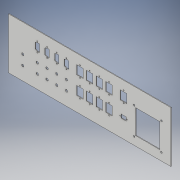
# Autodesk Inventor part: PDU_chassis
Saved by Autodesk Inventor 2017 (Build 210142000, 142)
## iProperties
Created: 2017-02-13
Part Number: PDU_chassis
Material: Generic
Document SubType Name: Modeling
Designer: Zara
Density: 1 g/cm^3
Appearance: Default
Author: Zara
Autodesk Inventor part; units mm, degrees
ref_plane "YZ Plane" through (0, 0, 0) normal (1, 0, 0) x (0, 1, 0)
ref_plane "XZ Plane" through (0, 0, 0) normal (0, 1, 0) x (-1, 0, 0)
ref_plane "XY Plane" through (0, 0, 0) normal (0, 0, 1) x (1, 0, 0)
sketch "Sketch1" plane through (0, 0, 0) normal (0, 0, 1) x (1, 0, 0)
  line L0 (-212.471, -66.7512) -> (212.471, -66.7512)
  line L1 (212.471, -66.7512) -> (212.471, 66.7512)
  line L2 (212.471, 66.7512) -> (-212.471, 66.7512)
  line L3 (-212.471, 66.7512) -> (-212.471, -66.7512)
  line L4 (-212.471, -66.7512) -> (212.471, 66.7512) construction
  line L5 (212.471, -66.7512) -> (-212.471, 66.7512) construction
  point P0 (0, 0)
  dimension "d0" = 424.942
  dimension "d1" = 133.5024
  constraints: 12 end point, 2 midpoint, 2 parallel, 1 horizontal, 1 perpendicular
  measures "d0" distance of L1.end L2.end
  measures "d1" distance of L0.end L1.end
extrude "pdu" add sketch "Sketch1" along normal blind 1.651
sketch "dsub9 sketch" plane through (0, 0, 1.651) normal (0, 0, 1) x (1, 0, 0)
  line L0 (-137.033, 41.9354) -> (-137.033, 16.9418) construction
  line L1 (-127.711, 29.4386) -> (-146.355, 29.4386) construction
  circle A0 centre (-137.033, 16.9418) radius 1.1303
  circle A1 centre (-137.033, 41.9354) radius 1.1303
  line L2 (-131.191, 37.8733) -> (-131.191, 21.0039)
  line L3 (-142.875, 36.1061) -> (-142.875, 22.7711)
  arc A2 (-133.7847, 18.9524) -> (-131.191, 21.0039) centre (-133.2992, 21.0039) ccw
  arc A3 (-142.875, 22.7711) -> (-141.2523, 20.7196) centre (-140.7668, 22.7711) ccw
  arc A4 (-141.1558, 38.1781) -> (-142.875, 36.1061) centre (-140.7668, 36.1061) ccw
  arc A5 (-131.191, 37.1546) -> (-133.6574, 39.5859) centre (-133.2684, 37.5139) ccw
  line L4 (-133.6574, 39.5859) -> (-141.1558, 38.1781)
  line L5 (-133.7847, 18.9524) -> (-141.2523, 20.7196)
  line L6 (209.423, 58.4962) -> (-209.423, 58.4962) construction
  line L7 (-209.423, 58.4962) -> (-209.423, -58.4962) construction
  line L8 (-209.423, -58.4962) -> (209.423, -58.4962) construction
  line L9 (209.423, -58.4962) -> (209.423, 58.4962) construction
  line L10 (212.471, 66.7512) -> (-212.471, 66.7512) construction
  line L11 (-212.471, -66.7512) -> (212.471, -66.7512) construction
  line L12 (-212.471, 66.7512) -> (-212.471, -66.7512) construction
  line L13 (212.471, -66.7512) -> (212.471, 66.7512) construction
  line L14 (-133.2992, 18.8957) -> (-149.9459, 18.8957) construction
  line L15 (-108.2574, 39.5859) -> (-115.7558, 38.1781)
  arc A6 (-105.791, 37.1546) -> (-108.2574, 39.5859) centre (-107.8684, 37.5139) ccw
  line L16 (-102.311, 29.4386) -> (-120.955, 29.4386) construction
  line L17 (-108.3847, 18.9524) -> (-115.8523, 20.7196)
  line L18 (-105.791, 37.8733) -> (-105.791, 21.0039)
  line L19 (-107.8992, 18.8957) -> (-124.5459, 18.8957) construction
  circle A7 centre (-111.633, 16.9418) radius 1.1303
  arc A8 (-108.3847, 18.9524) -> (-105.791, 21.0039) centre (-107.8992, 21.0039) ccw
  line L20 (-117.475, 36.1061) -> (-117.475, 22.7711)
  arc A9 (-117.475, 22.7711) -> (-115.8523, 20.7196) centre (-115.3668, 22.7711) ccw
  line L21 (-111.633, 41.9354) -> (-111.633, 16.9418) construction
  circle A10 centre (-111.633, 41.9354) radius 1.1303
  arc A11 (-115.7558, 38.1781) -> (-117.475, 36.1061) centre (-115.3668, 36.1061) ccw
  line L22 (-82.8574, 39.5859) -> (-90.3558, 38.1781)
  arc A12 (-80.391, 37.1546) -> (-82.8574, 39.5859) centre (-82.4684, 37.5139) ccw
  line L23 (-76.911, 29.4386) -> (-95.555, 29.4386) construction
  line L24 (-82.9847, 18.9524) -> (-90.4523, 20.7196)
  line L25 (-80.391, 37.8733) -> (-80.391, 21.0039)
  line L26 (-82.4992, 18.8957) -> (-99.1459, 18.8957) construction
  circle A13 centre (-86.233, 16.9418) radius 1.1303
  arc A14 (-82.9847, 18.9524) -> (-80.391, 21.0039) centre (-82.4992, 21.0039) ccw
  line L27 (-92.075, 36.1061) -> (-92.075, 22.7711)
  arc A15 (-92.075, 22.7711) -> (-90.4523, 20.7196) centre (-89.9668, 22.7711) ccw
  line L28 (-86.233, 41.9354) -> (-86.233, 16.9418) construction
  circle A16 centre (-86.233, 41.9354) radius 1.1303
  arc A17 (-90.3558, 38.1781) -> (-92.075, 36.1061) centre (-89.9668, 36.1061) ccw
  line L29 (-57.4574, 39.5859) -> (-64.9558, 38.1781)
  arc A18 (-54.991, 37.1546) -> (-57.4574, 39.5859) centre (-57.0684, 37.5139) ccw
  line L30 (-51.511, 29.4386) -> (-70.155, 29.4386) construction
  line L31 (-57.5847, 18.9524) -> (-65.0523, 20.7196)
  line L32 (-54.991, 37.8733) -> (-54.991, 21.0039)
  line L33 (-57.0992, 18.8957) -> (-73.7459, 18.8957) construction
  circle A19 centre (-60.833, 16.9418) radius 1.1303
  arc A20 (-57.5847, 18.9524) -> (-54.991, 21.0039) centre (-57.0992, 21.0039) ccw
  line L34 (-66.675, 36.1061) -> (-66.675, 22.7711)
  arc A21 (-66.675, 22.7711) -> (-65.0523, 20.7196) centre (-64.5668, 22.7711) ccw
  line L35 (-60.833, 41.9354) -> (-60.833, 16.9418) construction
  circle A22 centre (-60.833, 41.9354) radius 1.1303
  arc A23 (-64.9558, 38.1781) -> (-66.675, 36.1061) centre (-64.5668, 36.1061) ccw
  point P0 (0, 0)
  point P1 (-137.033, 29.4386)
  point P2 (-131.191, 29.4386)
  point P3 (-142.875, 29.4386)
  point P4 (-105.791, 29.4386)
  point P5 (-111.633, 29.4386)
  point P6 (-117.475, 29.4386)
  point P7 (-80.391, 29.4386)
  point P8 (-86.233, 29.4386)
  point P9 (-92.075, 29.4386)
  point P10 (-54.991, 29.4386)
  point P11 (-60.833, 29.4386)
  point P12 (-66.675, 29.4386)
  dimension "d24" = 38.1
  dimension "d205" = 25.4
  dimension "d208" = 25.4
  dimension "d4" = 2.2606
  dimension "d5" = 2.2606
  dimension "d6" = 24.9936
  dimension "d7" = 4.2164
  dimension "d8" = 4.2164
  dimension "d9" = 4.2164
  dimension "d10" = 4.2164
  dimension "d11" = 13.335
  dimension "d12" = 16.51
  dimension "d13" = 8.255
  dimension "d14" = 8.255
  dimension "d15" = 3.048
  dimension "d16" = 3.048
  dimension "d17" = 75.438
  dimension "d18" = 5.842
  dimension "d19" = 11.684
  dimension "d21" = 7.4985
  dimension "d165" = 37.3126
  dimension "d175" = 25.4
  constraints: 64 end point, 40 point on circle, 24 centre point, 12 point on line, 8 coincident, 8 tangent, 5 horizontal, 4 midpoint, 3 vertical, 2 parallel, 1 collinear, 1 perpendicular, 110 other
  measures "d4" diameter of A1
  measures "d5" diameter of A0
  measures "d6" distance of L0.start L0.end
  measures "d7" diameter of A2
  measures "d8" diameter of A3
  measures "d9" diameter of A5
  measures "d10" diameter of A4
  measures "d11" distance of A3.centre A4.centre
  measures "d12" distance of A2.centre A5.centre
  measures "d13" distance between parallel lines of L10 L6
  measures "d14" distance between parallel lines of L11 L8
  measures "d15" distance between parallel lines of L12 L7
  measures "d16" distance between parallel lines of L13 L9
  measures "d17" distance from line of L12 A0.centre
  measures "d18" distance from line of L2 A0.centre
  measures "d19" distance between parallel lines of L3 L2
  measures "d21" horizontal distance of A4.centre A5.centre
  measures "d165" distance between parallel lines of L10 L1
  measures "d175" distance of A4.centre A11.centre
sketch "CAT7 sketch" plane through (0, 0, 1.651) normal (0, 0, 1) x (1, 0, 0)
  line L0 (-34.124, 40.8686) -> (-16.979, 40.8686)
  line L1 (-16.979, 40.8686) -> (-16.979, 18.0086)
  line L2 (-16.979, 18.0086) -> (-34.124, 18.0086)
  line L3 (-34.124, 18.0086) -> (-34.124, 40.8686)
  line L4 (-43.4069, 29.4386) -> (12.6608, 29.4386) construction
  circle A0 centre (-25.5515, 43.942) radius 1.1303
  circle A1 centre (-25.5515, 14.9352) radius 1.1303
  line L5 (-25.5515, 43.942) -> (-25.5515, 14.9352) construction
  line L6 (-212.471, -66.7512) -> (212.471, -66.7512) construction
  line L7 (-212.471, 66.7512) -> (-212.471, -66.7512) construction
  line L8 (-34.124, -6.1722) -> (-16.979, -6.1722)
  line L9 (-16.979, -6.1722) -> (-16.979, -29.0322)
  line L10 (-16.979, -29.0322) -> (-34.124, -29.0322)
  line L11 (-34.124, -29.0322) -> (-34.124, -6.1722)
  circle A2 centre (-25.5515, -3.1073) radius 1.1303
  circle A3 centre (-25.5515, -32.1141) radius 1.1303
  line L12 (-25.5515, -3.1073) -> (-25.5515, -32.1141) construction
  circle A4 centre (-0.1515, 14.9352) radius 1.1303
  line L13 (8.421, 18.0086) -> (-8.724, 18.0086)
  line L14 (-18.0069, 29.4386) -> (38.0608, 29.4386) construction
  line L15 (8.421, 40.8686) -> (8.421, 18.0086)
  line L16 (-8.724, 40.8686) -> (8.421, 40.8686)
  line L17 (-8.724, 18.0086) -> (-8.724, 40.8686)
  line L18 (-0.1515, 43.942) -> (-0.1515, 14.9352) construction
  circle A5 centre (-0.1515, 43.942) radius 1.1303
  circle A6 centre (-0.1515, -3.1073) radius 1.1303
  line L19 (-8.724, -6.1722) -> (8.421, -6.1722)
  line L20 (8.421, -6.1722) -> (8.421, -29.0322)
  line L21 (8.421, -29.0322) -> (-8.724, -29.0322)
  line L22 (-8.724, -29.0322) -> (-8.724, -6.1722)
  line L23 (-0.1515, -3.1073) -> (-0.1515, -32.1141) construction
  circle A7 centre (-0.1515, -32.1141) radius 1.1303
  circle A8 centre (25.2485, 14.9352) radius 1.1303
  line L24 (33.821, 18.0086) -> (16.676, 18.0086)
  line L25 (7.3931, 29.4386) -> (63.4608, 29.4386) construction
  line L26 (33.821, 40.8686) -> (33.821, 18.0086)
  line L27 (16.676, 40.8686) -> (33.821, 40.8686)
  line L28 (16.676, 18.0086) -> (16.676, 40.8686)
  line L29 (25.2485, 43.942) -> (25.2485, 14.9352) construction
  circle A9 centre (25.2485, 43.942) radius 1.1303
  circle A10 centre (25.2485, -3.1073) radius 1.1303
  line L30 (16.676, -6.1722) -> (33.821, -6.1722)
  line L31 (33.821, -6.1722) -> (33.821, -29.0322)
  line L32 (33.821, -29.0322) -> (16.676, -29.0322)
  line L33 (16.676, -29.0322) -> (16.676, -6.1722)
  line L34 (25.2485, -3.1073) -> (25.2485, -32.1141) construction
  circle A11 centre (25.2485, -32.1141) radius 1.1303
  circle A12 centre (50.6485, 14.9352) radius 1.1303
  line L35 (59.221, 18.0086) -> (42.076, 18.0086)
  line L36 (32.7931, 29.4386) -> (88.8608, 29.4386) construction
  line L37 (59.221, 40.8686) -> (59.221, 18.0086)
  line L38 (42.076, 40.8686) -> (59.221, 40.8686)
  line L39 (42.076, 18.0086) -> (42.076, 40.8686)
  line L40 (50.6485, 43.942) -> (50.6485, 14.9352) construction
  circle A13 centre (50.6485, 43.942) radius 1.1303
  circle A14 centre (50.6485, -3.1073) radius 1.1303
  line L41 (42.076, -6.1722) -> (59.221, -6.1722)
  line L42 (59.221, -6.1722) -> (59.221, -29.0322)
  line L43 (59.221, -29.0322) -> (42.076, -29.0322)
  line L44 (42.076, -29.0322) -> (42.076, -6.1722)
  line L45 (50.6485, -3.1073) -> (50.6485, -32.1141) construction
  circle A15 centre (50.6485, -32.1141) radius 1.1303
  line L46 (32.9446, 29.4386) -> (89.0123, 29.4386) construction
  line L47 (80.176, 40.8686) -> (97.321, 40.8686)
  line L48 (97.321, 40.8686) -> (97.321, 18.0086)
  line L49 (97.321, 18.0086) -> (80.176, 18.0086)
  line L50 (80.176, 18.0086) -> (80.176, 40.8686)
  circle A16 centre (88.7485, 43.942) radius 1.1303
  circle A17 centre (88.7485, 14.9352) radius 1.1303
  line L51 (88.7485, 43.942) -> (88.7485, 14.9352) construction
  line L52 (212.471, 66.7512) -> (-212.471, 66.7512) projected
  line L53 (40.3437, -17.6022) -> (62.8778, -17.6022) construction
  point P0 (0, 0)
  point P1 (-34.124, 29.4386)
  point P2 (-25.5515, 40.8686)
  point P3 (-25.5515, 29.4386)
  point P4 (-25.5515, -6.1807)
  point P5 (-34.124, -17.6107)
  point P6 (-43.4069, -17.6107)
  point P7 (-25.5515, -17.6107)
  point P8 (25.4, 0)
  point P9 (-8.724, 29.4386)
  point P10 (-0.1515, 29.4386)
  point P11 (-0.1515, 40.8686)
  point P12 (-0.1515, -6.1807)
  point P13 (-18.0069, -17.6107)
  point P14 (-0.1515, -17.6107)
  point P15 (-8.724, -17.6107)
  point P16 (50.8, 0)
  point P17 (16.676, 29.4386)
  point P18 (25.2485, 29.4386)
  point P19 (25.2485, 40.8686)
  point P20 (25.2485, -6.1807)
  point P21 (7.3931, -17.6107)
  point P22 (25.2485, -17.6107)
  point P23 (16.676, -17.6107)
  point P24 (76.2, 0)
  point P25 (42.076, 29.4386)
  point P26 (50.6485, 29.4386)
  point P27 (50.6485, 40.8686)
  point P28 (50.6485, -6.1807)
  point P29 (32.7931, -17.6107)
  point P30 (50.6485, -17.6107)
  point P31 (42.076, -17.6107)
  point P32 (80.176, 29.4386)
  point P33 (88.7485, 40.8686)
  point P34 (88.7485, 29.4386)
  point P35 (98.2853, 29.4386)
  dimension "d47" = 22.86
  dimension "d48" = 17.145
  dimension "d49" = 2.2606
  dimension "d50" = 2.2606
  dimension "d51" = 29.0068
  dimension "d52" = 81.6864
  dimension "d53" = 186.9195
  dimension "d56" = 47.0408
  dimension "d132" = 25.4
  dimension "d146" = 22.86
  dimension "d147" = 17.145
  dimension "d148" = 2.2606
  dimension "d149" = 2.2606
  dimension "d150" = 29.0068
  dimension "d151" = 38.1
  dimension "d152" = 25.8826
  constraints: 94 end point, 18 centre point, 17 point on line, 8 horizontal, 6 midpoint, 4 parallel, 3 vertical, 2 perpendicular, 1 collinear, 119 other
  measures "d47" distance of L0.end L1.end
  measures "d48" distance of L1.end L2.end
  measures "d49" diameter of A0
  measures "d50" diameter of A1
  measures "d51" distance of L5.end L5.start
  measures "d52" distance from line of L6 L5.end
  measures "d53" distance from line of L7 L5.end
  measures "d56" distance of L0.start L11.end
  measures "d132" distance of point (0, 0) point (25.4, 0)
  measures "d146" distance of L47.end L49.start
  measures "d147" distance of L49.start L50.start
  measures "d148" diameter of A16
  measures "d149" diameter of A17
  measures "d150" distance of L51.end L51.start
  measures "d151" distance from line of L40 point (88.748, 29.439)
  measures "d152" distance between parallel lines of L52 L47
sketch "Sketch5" plane through (0, 0, 1.651) normal (0, 0, 1) x (1, 0, 0)
  line L0 (110.109, -53.1622) -> (193.929, -53.1622) construction
  line L1 (193.929, -53.1622) -> (193.929, 30.6578) construction
  line L2 (193.929, 30.6578) -> (110.109, 30.6578) construction
  line L3 (110.109, 30.6578) -> (110.109, -53.1622) construction
  line L4 (110.109, -53.1622) -> (193.929, 30.6578) construction
  line L5 (193.929, -53.1622) -> (110.109, 30.6578) construction
  line L6 (-212.471, 66.7512) -> (-212.471, -66.7512) projected
  line L7 (-212.471, -66.7512) -> (212.471, -66.7512) projected
  line L8 (120.269, -43.0022) -> (183.769, -43.0022)
  line L9 (183.769, -43.0022) -> (183.769, 20.4978)
  line L10 (183.769, 20.4978) -> (120.269, 20.4978)
  line L11 (120.269, 20.4978) -> (120.269, -43.0022)
  line L12 (120.269, -43.0022) -> (183.769, 20.4978) construction
  line L13 (183.769, -43.0022) -> (120.269, 20.4978) construction
  line L14 (116.332, -46.9392) -> (187.706, -46.9392) construction
  line L15 (187.706, -46.9392) -> (187.706, 24.4348) construction
  line L16 (187.706, 24.4348) -> (116.332, 24.4348) construction
  line L17 (116.332, 24.4348) -> (116.332, -46.9392) construction
  line L18 (116.332, -46.9392) -> (187.706, 24.4348) construction
  line L19 (187.706, -46.9392) -> (116.332, 24.4348) construction
  circle A0 centre (116.332, 24.4348) radius 2.2479
  circle A1 centre (187.706, 24.4348) radius 2.2479
  circle A2 centre (187.706, -46.9392) radius 2.2479
  circle A3 centre (116.332, -46.9392) radius 2.2479
  line L20 (120.269, -43.0022) -> (183.769, -43.0022)
  line L21 (183.769, -43.0022) -> (183.769, 20.4978)
  line L22 (183.769, 20.4978) -> (120.269, 20.4978)
  line L23 (120.269, 20.4978) -> (120.269, -43.0022)
  line L24 (120.269, -43.0022) -> (183.769, 20.4978) construction
  line L25 (183.769, -43.0022) -> (120.269, 20.4978) construction
  point P0 (0, 0)
  point P1 (152.019, -11.2522)
  point P2 (152.019, -11.2522)
  dimension "d63" = 83.82
  dimension "d64" = 83.82
  dimension "d65" = 322.58
  dimension "d66" = 13.589
  dimension "d67" = 63.5
  dimension "d68" = 63.5
  dimension "d69" = 71.374
  dimension "d70" = 4.4958
  dimension "d71" = 4.4958
  dimension "d72" = 4.4958
  dimension "d73" = 4.4958
  constraints: 48 end point, 10 midpoint, 8 parallel, 4 centre point, 4 horizontal, 4 perpendicular, 3 coincident, 1 point on line
  measures "d63" distance of L1.end L2.end
  measures "d64" distance of L2.end L0.start
  measures "d65" distance between parallel lines of L6 L3
  measures "d66" distance between parallel lines of L0 L7
  measures "d67" distance of L8.end L9.end
  measures "d68" distance of L8.start L8.end
  measures "d69" distance of L14.start L14.end
  measures "d70" diameter of A1
  measures "d71" diameter of A0
  measures "d72" diameter of A2
  measures "d73" diameter of A3
hole "airflow holes" at (187.706, 24.4348, 1.651) at (116.332, 24.4348, 1.651) at (116.332, -46.9392, 1.651) at (187.706, -46.9392, 1.651) direction (0, 0, -1) diameter 4.4958 end through all clearance for "Flat Head Machine Screw (82)" size "#8" standard "Ansi Unified Screw Threads"
sketch "Sketch7" plane through (0, 0, 1.651) normal (0, 0, 1) x (1, 0, 0)
  line L0 (110.109, -53.1622) -> (193.929, -53.1622) construction
  line L1 (193.929, -53.1622) -> (193.929, 30.6578) construction
  line L2 (193.929, 30.6578) -> (110.109, 30.6578) construction
  line L3 (110.109, 30.6578) -> (110.109, -53.1622) construction
  line L4 (110.109, -53.1622) -> (193.929, 30.6578) construction
  line L5 (193.929, -53.1622) -> (110.109, 30.6578) construction
  line L6 (-212.471, 66.7512) -> (-212.471, -66.7512)
  line L7 (-212.471, -66.7512) -> (212.471, -66.7512)
  line L8 (120.269, -43.0022) -> (183.769, -43.0022)
  line L9 (183.769, -43.0022) -> (183.769, 20.4978)
  line L10 (183.769, 20.4978) -> (120.269, 20.4978)
  line L11 (120.269, 20.4978) -> (120.269, -43.0022)
  line L12 (120.269, -43.0022) -> (183.769, 20.4978) construction
  line L13 (183.769, -43.0022) -> (120.269, 20.4978) construction
  line L14 (116.332, -46.9392) -> (187.706, -46.9392) construction
  line L15 (187.706, -46.9392) -> (187.706, 24.4348) construction
  line L16 (187.706, 24.4348) -> (116.332, 24.4348) construction
  line L17 (116.332, 24.4348) -> (116.332, -46.9392) construction
  line L18 (116.332, -46.9392) -> (187.706, 24.4348) construction
  line L19 (187.706, -46.9392) -> (116.332, 24.4348) construction
  circle A0 centre (116.332, 24.4348) radius 2.2479
  circle A1 centre (187.706, 24.4348) radius 2.2479
  circle A2 centre (187.706, -46.9392) radius 2.2479
  circle A3 centre (116.332, -46.9392) radius 2.2479
  line L20 (120.269, -43.0022) -> (183.769, -43.0022)
  line L21 (183.769, -43.0022) -> (183.769, 20.4978)
  line L22 (183.769, 20.4978) -> (120.269, 20.4978)
  line L23 (120.269, 20.4978) -> (120.269, -43.0022)
  line L24 (120.269, -43.0022) -> (183.769, 20.4978) construction
  line L25 (183.769, -43.0022) -> (120.269, 20.4978) construction
  point P0 (0, 0)
  point P1 (0, 0)
  point P2 (152.019, -11.2522)
  point P3 (152.019, -11.2522)
  dimension "d83" = 83.82
  dimension "d84" = 83.82
  dimension "d85" = 322.58
  dimension "d86" = 13.589
  dimension "d87" = 63.5
  dimension "d88" = 63.5
  dimension "d89" = 71.374
  dimension "d90" = 4.4958
  dimension "d91" = 4.4958
  dimension "d92" = 4.4958
  dimension "d93" = 4.4958
  constraints: 52 end point, 10 midpoint, 8 parallel, 4 centre point, 4 horizontal, 4 perpendicular, 3 coincident, 1 point on line
  measures "d83" distance of L1.end L2.end
  measures "d84" distance of L2.end L0.start
  measures "d85" distance between parallel lines of L6 L3
  measures "d86" distance between parallel lines of L0 L7
  measures "d87" distance of L8.end L9.end
  measures "d88" distance of L8.start L8.end
  measures "d89" distance of L14.start L14.end
  measures "d90" diameter of A1
  measures "d91" diameter of A0
  measures "d92" diameter of A2
  measures "d93" diameter of A3
extrude "airflow cutout" cut sketch "Sketch7" against normal through all contours L11 L10 L9 L8
hole "CAT7 holes" at (-25.5515, 43.942, 1.651) at (-25.5515, 14.9352, 1.651) at (-25.5515, -3.1073, 1.651) at (-25.5515, -32.1141, 1.651) at (-0.1515, 43.942, 1.651) at (-0.1515, 14.9352, 1.651) at (25.2485, 43.942, 1.651) at (25.2485, 14.9352, 1.651) at (50.6485, 43.942, 1.651) at (50.6485, 14.9352, 1.651) at (-0.1515, -3.1073, 1.651) at (-0.1515, -32.1141, 1.651) at (25.2485, -32.1141, 1.651) at (25.2485, -3.1073, 1.651) at (50.6485, -3.1073, 1.651) at (50.6485, -32.1141, 1.651) at (88.7485, 43.942, 1.651) at (88.7485, 14.9352, 1.651) direction (0, 0, -1) diameter 2.9464 end through all
extrude "CAT7 cutout" cut sketch "CAT7 sketch" against normal through all contours L0 L1 L2 L3 | L8 L9 L10 L11 | L13 L17 L16 L15 | L19 L20 L21 L22 | L24 L28 L27 L26 | L30 L31 L32 L33 | L35 L39 L38 L37 | L41 L42 L43 L44 | L47 L48 L49 L50
sketch "sma" plane through (0, 0, 1.651) normal (0, 0, 1) x (1, 0, 0)
  line L0 (-175.126, 2.9121) -> (-175.126, -16.382) construction
  line L1 (-183.1756, -6.2272) -> (-164.6712, -6.2272) construction
  arc A0 (-177.92, -7.7352) -> (-177.92, -4.7191) centre (-175.126, -6.2272) ccw
  line L2 (-177.92, -4.7191) -> (-177.92, -7.7352)
  line L3 (-137.033, 41.9354) -> (-137.033, 16.9418) construction
  line L4 (-137.026, 2.9121) -> (-137.026, -16.382) construction
  arc A1 (-139.82, -7.7352) -> (-139.82, -4.7191) centre (-137.026, -6.2272) ccw
  line L5 (-139.82, -4.7191) -> (-139.82, -7.7352)
  line L6 (-145.0756, -6.2272) -> (-126.5712, -6.2272) construction
  line L7 (-175.126, -22.4879) -> (-175.126, -41.782) construction
  arc A2 (-177.92, -33.1352) -> (-177.92, -30.1191) centre (-175.126, -31.6272) ccw
  line L8 (-177.92, -30.1191) -> (-177.92, -33.1352)
  line L9 (-183.1756, -31.6272) -> (-164.6712, -31.6272) construction
  line L10 (-137.026, -22.4879) -> (-137.026, -41.782) construction
  arc A3 (-139.82, -33.1352) -> (-139.82, -30.1191) centre (-137.026, -31.6272) ccw
  line L11 (-139.82, -30.1191) -> (-139.82, -33.1352)
  line L12 (-145.0756, -31.6272) -> (-126.5712, -31.6272) construction
  line L13 (-111.626, -22.4879) -> (-111.626, -41.782) construction
  line L14 (-114.42, -30.1191) -> (-114.42, -33.1352)
  arc A4 (-114.42, -33.1352) -> (-114.42, -30.1191) centre (-111.626, -31.6272) ccw
  line L15 (-114.42, -4.7191) -> (-114.42, -7.7352)
  line L16 (-119.6756, -31.6272) -> (-101.1712, -31.6272) construction
  arc A5 (-114.42, -7.7352) -> (-114.42, -4.7191) centre (-111.626, -6.2272) ccw
  line L17 (-119.6756, -6.2272) -> (-101.1712, -6.2272) construction
  line L18 (-86.226, -22.4879) -> (-86.226, -41.782) construction
  line L19 (-89.02, -30.1191) -> (-89.02, -33.1352)
  arc A6 (-89.02, -33.1352) -> (-89.02, -30.1191) centre (-86.226, -31.6272) ccw
  line L20 (-89.02, -4.7191) -> (-89.02, -7.7352)
  line L21 (-94.2756, -31.6272) -> (-75.7712, -31.6272) construction
  arc A7 (-89.02, -7.7352) -> (-89.02, -4.7191) centre (-86.226, -6.2272) ccw
  line L22 (-94.2756, -6.2272) -> (-75.7712, -6.2272) construction
  line L23 (-60.826, -22.4879) -> (-60.826, -41.782) construction
  line L24 (-63.62, -30.1191) -> (-63.62, -33.1352)
  arc A8 (-63.62, -33.1352) -> (-63.62, -30.1191) centre (-60.826, -31.6272) ccw
  line L25 (-63.62, -4.7191) -> (-63.62, -7.7352)
  line L26 (-68.8756, -31.6272) -> (-50.3712, -31.6272) construction
  arc A9 (-63.62, -7.7352) -> (-63.62, -4.7191) centre (-60.826, -6.2272) ccw
  line L27 (-68.8756, -6.2272) -> (-50.3712, -6.2272) construction
  point P0 (0, 0)
  point P1 (-171.951, -6.2272)
  point P2 (-133.851, -6.2272)
  point P3 (-171.951, -31.6272)
  point P4 (-133.851, -31.6272)
  point P5 (-108.451, -31.6272)
  point P6 (-111.626, -16.382)
  point P7 (-108.451, -6.2272)
  point P8 (-83.051, -31.6272)
  point P9 (-86.226, -16.382)
  point P10 (-83.051, -6.2272)
  point P11 (-57.651, -31.6272)
  point P12 (-60.826, -16.382)
  point P13 (-57.651, -6.2272)
  dimension "d208" = 25.4
  dimension "d123" = 6.35
  dimension "d124" = 5.969
  dimension "d191" = 38.1
  dimension "d198" = 25.4
  dimension "d205" = 25.4
  constraints: 54 end point, 30 point on circle, 27 point on line, 10 centre point, 3 collinear, 3 horizontal, 3 vertical, 99 other
  measures "d123" diameter of A0
  measures "d124" distance from line of point (-171.951, -6.227) L2
  measures "d191" distance of L0.start L4.start
  measures "d198" distance of L0.start L7.start
  measures "d205" distance of L12.start L16.start
extrude "sma cutouts" cut sketch "sma" against normal through all
sketch "sc/sc" plane through (0, 0, 1.651) normal (0, 0, 1) x (1, 0, 0)
  line L0 (82.0175, -12.9032) -> (95.4795, -12.9032)
  line L1 (95.4795, -12.9032) -> (95.4795, -22.3012)
  line L2 (95.4795, -22.3012) -> (82.0175, -22.3012)
  line L3 (82.0175, -22.3012) -> (82.0175, -12.9032)
  line L4 (82.0175, -12.9032) -> (95.4795, -22.3012) construction
  line L5 (95.4795, -12.9032) -> (82.0175, -22.3012) construction
  line L6 (79.7485, -17.6022) -> (97.7485, -17.6022) construction
  arc A0 (-177.92, -7.7352) -> (-177.92, -4.7191) centre (-175.126, -6.2272) ccw projected
  line L7 (-177.92, -7.7352) -> (-177.92, -4.7191) projected
  line L8 (42.076, 18.0086) -> (42.076, 40.8686) projected
  line L9 (42.076, 40.8686) -> (59.221, 40.8686) projected
  line L10 (59.221, 40.8686) -> (59.221, 18.0086) projected
  line L11 (59.221, 18.0086) -> (42.076, 18.0086) projected
  line L12 (16.676, 18.0086) -> (16.676, 40.8686) projected
  line L13 (16.676, 40.8686) -> (33.821, 40.8686) projected
  line L14 (33.821, 40.8686) -> (33.821, 18.0086) projected
  line L15 (33.821, 18.0086) -> (16.676, 18.0086) projected
  line L16 (-8.724, 18.0086) -> (-8.724, 40.8686) projected
  line L17 (-8.724, 40.8686) -> (8.421, 40.8686) projected
  line L18 (8.421, 40.8686) -> (8.421, 18.0086) projected
  line L19 (8.421, 18.0086) -> (-8.724, 18.0086) projected
  line L20 (-34.124, 18.0086) -> (-34.124, 40.8686) projected
  line L21 (-34.124, 40.8686) -> (-16.979, 40.8686) projected
  line L22 (-16.979, 40.8686) -> (-16.979, 18.0086) projected
  line L23 (-16.979, 18.0086) -> (-34.124, 18.0086) projected
  line L24 (-34.124, -29.0322) -> (-34.124, -6.1722) projected
  line L25 (-34.124, -6.1722) -> (-16.979, -6.1722) projected
  line L26 (-16.979, -6.1722) -> (-16.979, -29.0322) projected
  line L27 (-16.979, -29.0322) -> (-34.124, -29.0322) projected
  line L28 (-8.724, -29.0322) -> (-8.724, -6.1722) projected
  line L29 (-8.724, -6.1722) -> (8.421, -6.1722) projected
  line L30 (8.421, -6.1722) -> (8.421, -29.0322) projected
  line L31 (8.421, -29.0322) -> (-8.724, -29.0322) projected
  line L32 (16.676, -29.0322) -> (16.676, -6.1722) projected
  line L33 (16.676, -6.1722) -> (33.821, -6.1722) projected
  line L34 (33.821, -6.1722) -> (33.821, -29.0322) projected
  line L35 (33.821, -29.0322) -> (16.676, -29.0322) projected
  line L36 (42.076, -29.0322) -> (42.076, -6.1722) projected
  line L37 (42.076, -6.1722) -> (59.221, -6.1722) projected
  line L38 (59.221, -6.1722) -> (59.221, -29.0322) projected
  line L39 (59.221, -29.0322) -> (42.076, -29.0322) projected
  circle A1 centre (50.6485, -3.1073) radius 1.4732 projected
  circle A2 centre (25.2485, -32.1141) radius 1.4732 projected
  circle A3 centre (-0.1515, -3.1073) radius 1.4732 projected
  circle A4 centre (50.6485, 43.942) radius 1.4732 projected
  circle A5 centre (25.2485, 43.942) radius 1.4732 projected
  circle A6 centre (-0.1515, 43.942) radius 1.4732 projected
  circle A7 centre (-25.5515, -3.1073) radius 1.4732 projected
  circle A8 centre (-25.5515, 43.942) radius 1.4732 projected
  circle A9 centre (-25.5515, 14.9352) radius 1.4732 projected
  circle A10 centre (-25.5515, -32.1141) radius 1.4732 projected
  circle A11 centre (-0.1515, 14.9352) radius 1.4732 projected
  circle A12 centre (25.2485, 14.9352) radius 1.4732 projected
  circle A13 centre (50.6485, 14.9352) radius 1.4732 projected
  circle A14 centre (-0.1515, -32.1141) radius 1.4732 projected
  circle A15 centre (25.2485, -3.1073) radius 1.4732 projected
  circle A16 centre (50.6485, -32.1141) radius 1.4732 projected
  line L40 (120.269, -43.0022) -> (120.269, 20.4978) projected
  line L41 (120.269, 20.4978) -> (183.769, 20.4978) projected
  line L42 (183.769, 20.4978) -> (183.769, -43.0022) projected
  line L43 (183.769, -43.0022) -> (120.269, -43.0022) projected
  circle A17 centre (116.332, -46.9392) radius 2.2479 projected
  circle A18 centre (187.706, 24.4348) radius 2.2479 projected
  circle A19 centre (116.332, 24.4348) radius 2.2479 projected
  circle A20 centre (187.706, -46.9392) radius 2.2479 projected
  line L44 (-212.471, -66.7512) -> (212.471, -66.7512) projected
  line L45 (212.471, -66.7512) -> (212.471, 66.7512) projected
  line L46 (212.471, 66.7512) -> (-212.471, 66.7512) projected
  line L47 (-212.471, 66.7512) -> (-212.471, -66.7512) projected
  line L48 (88.7485, 43.942) -> (88.7485, 14.9352) construction
  line L49 (80.176, 40.8686) -> (97.321, 40.8686) projected
  line L50 (80.176, 18.0086) -> (80.176, 40.8686) projected
  line L51 (97.321, 18.0086) -> (80.176, 18.0086) projected
  line L52 (97.321, 40.8686) -> (97.321, 18.0086) projected
  circle A21 centre (88.7485, 14.9352) radius 1.1303 projected
  line L53 (88.7485, -17.6022) -> (88.7485, -9.8781) construction
  line L54 (40.3437, -17.6022) -> (62.8778, -17.6022) construction
  point P0 (0, 0)
  point P1 (88.7485, -17.6022)
  dimension "d153" = 13.462
  dimension "d154" = 9.398
  dimension "d155" = 18
  constraints: 16 end point, 4 midpoint, 2 coincident, 2 collinear, 2 horizontal, 2 parallel, 1 perpendicular, 1 vertical
  measures "d153" distance of L0.start L0.end
  measures "d154" distance of L0.end L1.end
  measures "d155" distance of L6.start L6.end
hole "sc/sc holes" at (97.7485, -17.6022, 1.651) at (79.7485, -17.6022, 1.651) direction (0, 0, -1) diameter 2.3876 end through all clearance for "Countersunk Flat Head Screw ISO 2009/7046" size "M2" standard "ISO"
extrude "sc cutout" cut sketch "sc/sc" against normal blind 25.4 contours L0 L1 L2 L3
extrude "Extrusion12" cut sketch "dsub9 sketch" against normal blind 25.4 contours L2 A2 L5 A3 L3 A4 L4 A5 | A6 L18 A8 L17 A9 L20 A11 L15 | A12 L25 A14 L24 A15 L27 A17 L22 | A18 L32 A20 L31 A21 L34 A23 L29
hole "Hole6" at (-137.033, 41.9354, 1.651) at (-137.033, 16.9418, 1.651) at (-111.633, 41.9354, 1.651) at (-111.633, 16.9418, 1.651) at (-86.233, 16.9418, 1.651) at (-86.233, 41.9354, 1.651) at (-60.833, 16.9418, 1.651) at (-60.833, 41.9354, 1.651) direction (0, 0, -1) diameter 2.9464 end through all clearance for "Flat Head Machine Screw (82)" size "#4" standard "Ansi Unified Screw Threads"
body "Solid1"
